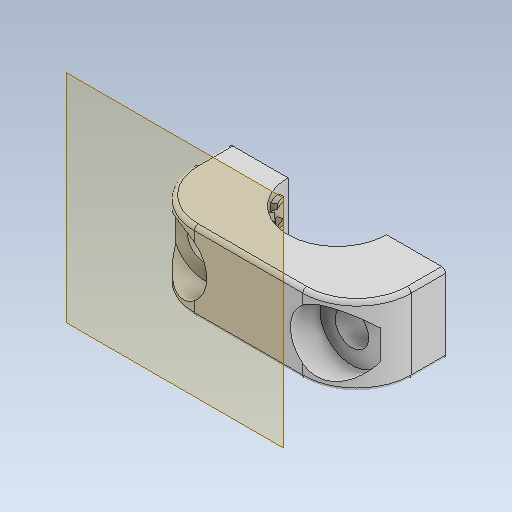
# Autodesk Inventor part: Extruder Cable Clamp
Saved by Autodesk Inventor 2023 (Build 270158000, 158)
## iProperties
Created: 2019-11-15
Part Number: Extruder Cable Clamp
Material: Generic
Document SubType Name: Modeling
Designer: pepd9
Density: 1 g/cm^3
Appearance: Default
Author: pepd9
Autodesk Inventor part; units mm, degrees
ref_plane "YZ Plane" through (0, 0, 0) normal (1, 0, 0) x (0, 1, 0)
ref_plane "XZ Plane" through (0, 0, 0) normal (0, 1, 0) x (-1, 0, 0)
ref_plane "XY Plane" through (0, 0, 0) normal (0, 0, 1) x (1, 0, 0)
sketch "Sketch1" plane through (0, 0, 0) normal (0, 1, 0) x (-1, 0, 0)
  arc A0 (-10, 0) -> (0, 0) centre (-5, 0) ccw projected
  line L0 (6, 0) -> (0, 0) projected
  line L1 (-10, 0) -> (-12, 0) projected
  circle A1 centre (-5, 0) radius 5
  line L2 (-12, 0) -> (6, 0)
  line L3 (6, 0) -> (6, 9)
  line L4 (6, 9) -> (-12, 9)
  line L5 (-12, 9) -> (-12, 0)
  point P0 (0, 0)
  dimension "d0" = 9
  constraints: 8 end point, 2 parallel, 1 coincident, 1 horizontal, 1 perpendicular, 1 point on line, 3 other
  measures "d0" distance of L2.end L3.end
ref_plane "Work Plane1" through (-6, -8, -5) normal (0, -1, 0) x (1, 0, 0)
extrude "Extrusion1" add sketch "Sketch1" against normal up to surface (8 mm away) contours L1 L5 L4 L3 L0 A1
fillet "Fillet2" radius 5.5 2 edges at (-6, -4, 9) (12, -4, 9)
ref_plane "Work Plane2" through (5, -7.5, 0) normal (0, -1, 0) x (1, 0, 0)
sketch "Sketch3" plane through (5, -7.5, 0) normal (0, -1, 0) x (1, 0, 0)
  arc A0 (5, 0) -> (-5, 0) centre (0, 0) ccw projected
  circle A1 centre (0, 0) radius 4.5
  line L0 (-5, 0) -> (-4.5, 0)
  line L1 (-4.8547, 1.1966) -> (-4.3692, 1.0769)
  line L2 (-4.4273, 2.3236) -> (-3.9846, 2.0913)
  line L3 (-3.7426, 3.3156) -> (-3.3683, 2.9841)
  line L4 (-2.8403, 4.1149) -> (-2.5563, 3.7034)
  line L5 (-1.773, 4.6751) -> (-1.5957, 4.2076)
  line L6 (-0.6027, 4.9635) -> (-0.5424, 4.4672)
  line L7 (0.6027, 4.9635) -> (0.5424, 4.4672)
  line L8 (1.773, 4.6751) -> (1.5957, 4.2076)
  line L9 (2.8403, 4.1149) -> (2.5563, 3.7034)
  line L10 (3.7426, 3.3156) -> (3.3683, 2.9841)
  line L11 (4.4273, 2.3236) -> (3.9846, 2.0913)
  line L12 (4.8547, 1.1966) -> (4.3692, 1.0769)
  line L13 (5, 0) -> (4.5, 0)
  point P0 (-3.9846, 2.0913)
  point P1 (-4.4273, 2.3236)
  point P2 (-2.5563, 3.7034)
  point P3 (-2.8403, 4.1149)
  point P4 (-3.7426, 3.3156)
  point P5 (-3.3683, 2.9841)
  point P6 (-0.5424, 4.4672)
  point P7 (-1.5957, 4.2076)
  point P8 (1.5957, 4.2076)
  point P9 (1.773, 4.6751)
  point P10 (0.6027, 4.9635)
  point P11 (0.5424, 4.4672)
  point P12 (3.3683, 2.9841)
  point P13 (3.7426, 3.3156)
  point P14 (2.8403, 4.1149)
  point P15 (2.5563, 3.7034)
  point P16 (3.9846, 2.0913)
  dimension "d13" = 9
  dimension "d16" = 180
  constraints: 28 end point, 1 coincident, 1 horizontal, 43 other
extrude "Extrusion2" add sketch "Sketch3" against normal blind 0.75 contours L12 A1 L11 A0 | L10 A1 L9 A0 | L1 A0 L2 A1 | L8 A1 L7 A0 | L3 A0 L4 A1 | L6 A1 L5 A0
pattern_linear "Rectangular Pattern1" count 4 spacing 2 along (0, 1, 0) of "Extrusion2"
ref_plane "Work Plane3" through (5, -6, 0) normal (0, -1, 0) x (1, 0, 0)
chamfer "Chamfer2" distance 0.5 angle 30 1 edges at (7.9841, -7.5, 3.3683) measured on face at (8.0504, -7.5, 3.4431)
chamfer "Chamfer3" distance 0.5 angle 30 1 edges at (9.2076, -7.5, 1.5957) measured on face at (9.3011, -7.5, 1.6312)
chamfer "Chamfer4" distance 0.5 angle 30 1 edges at (6.0769, -7.5, 4.3692) measured on face at (6.1009, -7.5, 4.4663)
chamfer "Chamfer5" distance 0.5 angle 30 1 edges at (3.9231, -7.5, 4.3692) measured on face at (3.8991, -7.5, 4.4663)
chamfer "Chamfer6" distance 0.5 angle 30 1 edges at (2.0159, -7.5, 3.3683) measured on face at (1.9496, -7.5, 3.4431)
chamfer "Chamfer7" distance 0.5 angle 30 1 edges at (0.7924, -7.5, 1.5957) measured on face at (0.6989, -7.5, 1.6312)
chamfer "Chamfer8" distance 0.5 angle 30 1 edges at (0.7924, -5.5, 1.5957) measured on face at (0.6989, -5.5, 1.6312)
chamfer "Chamfer9" distance 0.5 angle 30 1 edges at (2.0159, -5.5, 3.3683) measured on face at (1.9496, -5.5, 3.4431)
chamfer "Chamfer10" distance 0.5 angle 30 1 edges at (3.9231, -5.5, 4.3692) measured on face at (3.8991, -5.5, 4.4663)
chamfer "Chamfer11" distance 0.5 angle 30 1 edges at (6.0769, -5.5, 4.3692) measured on face at (6.1009, -5.5, 4.4663)
chamfer "Chamfer12" distance 0.5 angle 30 1 edges at (7.9841, -5.5, 3.3683) measured on face at (8.0504, -5.5, 3.4431)
chamfer "Chamfer13" distance 0.5 angle 30 1 edges at (9.2076, -5.5, 1.5957) measured on face at (9.3011, -5.5, 1.6312)
chamfer "Chamfer14" distance 0.5 angle 30 1 edges at (9.2076, -3.5, 1.5957) measured on face at (9.3011, -3.5, 1.6312)
chamfer "Chamfer15" distance 0.5 angle 30 1 edges at (7.9841, -3.5, 3.3683) measured on face at (8.0504, -3.5, 3.4431)
chamfer "Chamfer16" distance 0.5 angle 30 1 edges at (6.0769, -3.5, 4.3692) measured on face at (6.1009, -3.5, 4.4663)
chamfer "Chamfer17" distance 0.5 angle 30 1 edges at (3.9231, -3.5, 4.3692) measured on face at (3.8991, -3.5, 4.4663)
chamfer "Chamfer18" distance 0.5 angle 30 1 edges at (2.0159, -3.5, 3.3683) measured on face at (1.9496, -3.5, 3.4431)
chamfer "Chamfer19" distance 0.5 angle 30 1 edges at (0.7924, -3.5, 1.5957) measured on face at (0.6989, -3.5, 1.6312)
chamfer "Chamfer20" distance 0.5 angle 30 1 edges at (0.7924, -1.5, 1.5957) measured on face at (0.6989, -1.5, 1.6312)
chamfer "Chamfer21" distance 0.5 angle 30 1 edges at (2.0159, -1.5, 3.3683) measured on face at (1.9496, -1.5, 3.4431)
chamfer "Chamfer22" distance 0.5 angle 30 1 edges at (3.9231, -1.5, 4.3692) measured on face at (3.8991, -1.5, 4.4663)
chamfer "Chamfer23" distance 0.5 angle 30 1 edges at (6.0769, -1.5, 4.3692) measured on face at (6.1009, -1.5, 4.4663)
chamfer "Chamfer24" distance 0.5 angle 30 1 edges at (7.9841, -1.5, 3.3683) measured on face at (8.0504, -1.5, 3.4431)
chamfer "Chamfer25" distance 0.5 angle 30 1 edges at (9.2076, -1.5, 1.5957) measured on face at (9.3011, -1.5, 1.6312)
move faces "Move1" translate (4, 0, 0) faces at (12, -2.6667, 2.3333)
ref_plane "Work Plane4" through (-2.5, -4, 9) normal (0, 0, 1) x (1, 0, 0)
sketch "Sketch5" plane through (-2.5, -4, 9) normal (0, 0, 1) x (1, 0, 0)
  circle A0 centre (15, 0) radius 1.7 projected
  circle A1 centre (0, 0) radius 1.95 projected
  point P0 (2.5, 4)
hole "Hole2" at (12.5, -4, 9) at (-2.5, -4, 9) direction (0, 0, -1) diameter 3.4 end through all counterbore diameter 6.5 counterbore depth 3 clearance for "Socket Head Cap Screw" size "M3" standard "Ansi Metric M Profile"
fillet "Fillet3" radius 0.4 10 edges at (-4.3891, 0, 7.3891) (5, 0, 9) (14.3891, 0, 7.3891) (16, 0, 1.75) (-6, 0, 1.75) (-4.3891, -8, 7.3891) (5, -8, 9) (14.3891, -8, 7.3891) (16, -8, 1.75) (-6, -8, 1.75)
body "Solid1"
